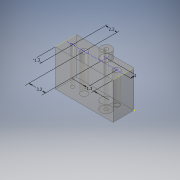
# Autodesk Inventor part: BOt
Saved by Autodesk Inventor 2019 (Build 230136000, 136)
## iProperties
Created: 2019-02-01
Part Number: BOt
Material: 일반
Document SubType Name: Modeling
Designer: Jeong Ji Hoon
Density: 1 g/cm^3
Appearance: 연회색 반사
Author: Jeong Ji Hoon
## iProperties of the stored document Bot_3D 인쇄.ipt
Created: 2019-02-07
Part Number: Bot_3D 인쇄
Material: 일반
Document SubType Name: Modeling
Designer: Jeong Ji Hoon
Density: 1 g/cm^3
Appearance: 기본값
Author: Jeong Ji Hoon
Autodesk Inventor part; units mm, degrees
ref_plane "YZ Plane" through (0, 0, 0) normal (1, 0, 0) x (0, 1, 0)
ref_plane "XZ Plane" through (0, 0, 0) normal (0, 1, 0) x (-1, 0, 0)
ref_plane "XY Plane" through (0, 0, 0) normal (0, 0, 1) x (1, 0, 0)
sketch "스케치1" plane through (0, 0, 0) normal (0, 1, 0) x (-1, 0, 0)
  line L0 (0, 0) -> (11, 0)
  line L1 (11, 0) -> (11, -4)
  line L2 (11, -4) -> (0, -4)
  line L3 (0, -4) -> (0, 0)
  dimension "d0" = 11
  dimension "d1" = 4
  constraints: 8 end point, 2 parallel, 1 horizontal, 1 perpendicular
  measures "d0" distance of L1.end L2.end
  measures "d1" distance of L0.end L1.end
extrude "돌출1" add sketch "스케치1" along normal blind 7
sketch "스케치2" plane through (0, 7, 0) normal (0, 1, 0) x (1, 0, 0)
  line L0 (0, 0) -> (0, 4) construction
  line L1 (0, 2) -> (-11, 2) construction
  line L2 (-11, 4) -> (-11, 0) construction
  point P0 (-1.3, 2)
  point P1 (-4.3, 2)
  point P2 (-7.5, 2)
  point P3 (-9.7, 2)
  point P4 (-4.3, 3)
  dimension "d59" = 1.3
  dimension "d60" = 2.2
  dimension "d61" = 3.2
  dimension "d62" = 1.3
  dimension "d69" = 1
  constraints: 4 point on line, 2 end point, 2 midpoint, 1 vertical alignment
  measures "d59" distance from line of L2 point (-9.7, 2)
  measures "d60" distance of point (-9.7, 2) point (-7.5, 2)
  measures "d61" distance of point (-4.3, 2) point (-7.5, 2)
  measures "d62" distance from line of L0 point (-1.3, 2)
  measures "d69" distance from line of L1 point (-4.3, 3)
hole "구멍1" at (-9.7, 7, -2) direction (0, -1, 0) diameter 0.65 end through all
hole "구멍2" at (-7.5, 7, -2) direction (0, -1, 0) diameter 1.3 end through all
hole "구멍3" at (-4.3, 7, -3) direction (0, -1, 0) diameter 0.67 end through all
hole "구멍4" at (-1.3, 7, -2) direction (0, -1, 0) diameter 1 depth 5.8 tip angle 90 countersink diameter 1.3 countersink angle 3
sketch "스케치3" plane through (0, 7, 0) normal (0, 1, 0) x (1, 0, 0)
  circle A0 centre (-4.3, 3) radius 1
  circle A1 centre (-4.3, 3) radius 0.335 projected
  point P0 (0, 0)
  point P1 (-4.3, 2)
  dimension "d50" = 2
  constraints: 1 centre point, 1 coincident
  measures "d50" diameter of A0
extrude "돌출2" add sketch "스케치3" along normal blind 1.5
sketch "스케치4" plane through (0, 0, 0) normal (0, -1, 0) x (1, 0, 0)
  circle A0 centre (-4.3, -3) radius 1
  circle A1 centre (-4.3, -3) radius 0.335 projected
  point P0 (0, 0)
  point P1 (-4.3, -2)
  dimension "d53" = 2
  constraints: 1 centre point, 1 coincident
  measures "d53" diameter of A0
extrude "돌출3" add sketch "스케치4" along normal blind 1.5
sketch "스케치5" plane through (0, 0, -4) normal (0, 0, -1) x (-1, 0, 0)
  point P0 (0, 0)
equation "\"d8\" = G23_F"
equation "\"d15\" = Screw_F"
equation "\"d22\" = G23_M"
equation "\"G23_F\" = 0.65"
equation "\"G23_M\" = 0.67"
equation "\"Screw_F\" = 1.3"
equation "\"Screw_M\" = 1.6"
